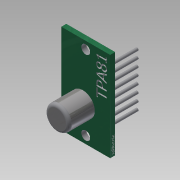
# Autodesk Inventor part: TPA81
Saved by Autodesk Inventor 2015 SP1 (Build 190203100, 203)
## iProperties
Created: 2015-01-28
Part Number: TPA81
Material: Generic
Document SubType Name: Modeling
Designer: Rafi Kurnia Putra
Density: 1 g/cm^3
Appearance: Default
Mass: 1.33618 g
Surface Area: 17.4789 cm^2
Volume: 1.33618 cm^3
Author: Rafi Kurnia Putra
Autodesk Inventor part; units mm, degrees
sketch "Sketch1" plane through (0, 0, 0) normal (0, 1, 0) x (-1, 0, 0)
  line L0 (8.3, 15.2) -> (-8.3, 15.2)
  line L1 (-8.3, 15.2) -> (-8.3, -15.2)
  line L2 (-8.3, -15.2) -> (8.3, -15.2)
  line L3 (8.3, -15.2) -> (8.3, 15.2)
  circle A0 centre (0, -12.66) radius 1.5
  circle A1 centre (0, 12.66) radius 1.5
  circle A2 centre (1, 3.9) radius 4.09
  point P0 (0, 0)
  dimension "d0" = 16.6
  dimension "d1" = 30.4
  dimension "d2" = 3
  dimension "d3" = 3
  dimension "d4" = 2.54
  dimension "d5" = 2.54
  dimension "d6" = 8.18
  dimension "d7" = 7.3
  dimension "d8" = 11.3
  constraints: 8 end point, 3 centre point, 2 parallel, 1 horizontal, 1 perpendicular
  measures "d0" distance of L2.end L1.end
  measures "d1" distance of L1.end L0.end
  measures "d2" diameter of A0
  measures "d3" diameter of A1
  measures "d4" distance from line of A1.centre L0
  measures "d5" distance from line of A0.centre L2
  measures "d6" diameter of A2
  measures "d7" distance from line of A2.centre L3
  measures "d8" distance from line of L0 A2.centre
extrude "Extrusion1" add sketch "Sketch1" along normal blind 1.7
extrude "Extrusion2" add sketch "Sketch1" along normal blind 10.5 contours A2
fillet "Fillet1" radius 1 1 edges at (3.09, 10.5, 3.9)
sketch "Sketch2" plane through (0, 1.7, 0) normal (0, 1, 0) x (1, 0, 0)
  line L0 (3.3822, -3.3689) -> (3.3822, 14.1226) construction
  line L1 (3.3822, 14.1226) -> (7.041, 14.1226) construction
  line L2 (7.041, 14.1226) -> (7.041, -3.3689) construction
  line L3 (7.041, -3.3689) -> (3.3822, -3.3689) construction
  point P0 (0, 0)
  constraints: 2 other
sketch "Sketch3" plane through (0, 0, 0) normal (0, -1, 0) x (1, 0, 0)
  circle A0 centre (5.76, 7.98) radius 0.5
  circle A1 centre (5.76, 5.44) radius 0.5
  circle A2 centre (5.76, 2.9) radius 0.5
  circle A3 centre (5.76, -2.18) radius 0.5
  circle A4 centre (5.76, -4.72) radius 0.5
  circle A5 centre (5.76, -7.26) radius 0.5
  circle A6 centre (5.76, -9.8) radius 0.5
  line L0 (8.3, 15.2) -> (8.3, -15.2) projected
  line L1 (8.3, -15.2) -> (-8.3, -15.2) projected
  circle A7 centre (5.76, 0.36) radius 0.5
  point P0 (0, 0)
  dimension "d30" = 1
  dimension "d31" = 1
  dimension "d32" = 1
  dimension "d33" = 1
  dimension "d34" = 1
  dimension "d35" = 1
  dimension "d36" = 1
  dimension "d37" = 2.54
  dimension "d38" = 2.54
  dimension "d39" = 2.54
  dimension "d40" = 2.54
  dimension "d41" = 2.54
  dimension "d43" = 2.54
  dimension "d44" = 5.4
  dimension "d47" = 1
  dimension "d48" = 2.54
  dimension "d49" = 2.54
  constraints: 8 centre point, 1 vertical alignment
  measures "d30" diameter of A0
  measures "d31" diameter of A1
  measures "d32" diameter of A2
  measures "d33" diameter of A3
  measures "d34" diameter of A4
  measures "d35" diameter of A5
  measures "d36" diameter of A6
  measures "d37" distance of A1.centre A0.centre
  measures "d38" distance of A1.centre A2.centre
  measures "d39" distance of A4.centre A3.centre
  measures "d40" distance of A4.centre A5.centre
  measures "d41" distance of A5.centre A6.centre
  measures "d43" distance from line of A6.centre L0
  measures "d44" distance from line of A6.centre L1
  measures "d47" diameter of A7
  measures "d48" distance of A7.centre A2.centre
  measures "d49" distance of A3.centre A7.centre
extrude "Extrusion3" add sketch "Sketch3" along normal blind 10 contours A0 | A1 | A2 | A3 | A4 | A5 | A6
extrude "Extrusion4" add sketch "Sketch3" along normal blind 10 contours A7
sketch "Sketch4" plane through (0, 1.7, 0) normal (0, 1, 0) x (1, 0, 0)
  line L0 (3.5532, 0.6031) -> (3.5532, 14.2089) construction
  line L1 (3.5532, 14.2089) -> (12.8953, 14.2089) construction
  line L2 (12.8953, 14.2089) -> (12.8953, 0.6031) construction
  line L3 (12.8953, 0.6031) -> (3.5532, 0.6031) construction
  line L4 (7.1326, 1.7745) -> (4.0467, 1.7745)
  line L5 (4.0467, 1.7745) -> (4.0467, 0.6003)
  line L6 (4.0467, 0.6003) -> (3.6326, 0.6003)
  line L7 (3.6326, 0.6003) -> (3.6326, 3.4139)
  line L8 (3.6326, 3.4139) -> (4.0467, 3.4139)
  line L9 (4.0467, 3.4139) -> (4.0467, 2.2397)
  line L10 (4.0467, 2.2397) -> (7.1326, 2.2397)
  line L11 (7.1326, 2.2397) -> (7.1326, 1.7745)
  spline S0 degree 2 poles (4.6877, 5.9807) (4.9146, 5.9807) (5.3231, 5.8191) (5.4649, 5.6744) knots 0 0 0 1 2 2 2
  spline S1 degree 2 poles (5.4649, 5.6744) (5.6436, 5.4929) (5.8279, 5.0022) (5.8279, 4.6278) knots 0 0 0 1 2 2 2
  line L12 (5.8279, 4.6278) -> (5.8279, 4.2336)
  line L13 (5.8279, 4.2336) -> (7.1326, 4.2336)
  line L14 (7.1326, 4.2336) -> (7.1326, 3.7684)
  line L15 (7.1326, 3.7684) -> (3.6326, 3.7684)
  line L16 (3.6326, 3.7684) -> (3.6326, 4.6477)
  spline S2 degree 2 poles (3.6326, 4.6477) (3.6326, 4.9597) (3.7347, 5.3965) (3.851, 5.5638) knots 0 0 0 1 2 2 2
  spline S3 degree 2 poles (3.851, 5.5638) (3.9843, 5.7595) (4.3956, 5.9807) (4.6877, 5.9807) knots 0 0 0 1 2 2 2
  spline S4 degree 2 poles (4.7019, 5.4957) (4.5204, 5.4957) (4.2538, 5.3709) (4.1687, 5.2433) knots 0 0 0 1 2 2 2
  spline S5 degree 2 poles (4.1687, 5.2433) (4.0949, 5.1327) (4.0354, 4.8377) (4.0354, 4.6193) knots 0 0 0 1 2 2 2
  line L17 (4.0354, 4.6193) -> (4.0354, 4.2336)
  line L18 (4.0354, 4.2336) -> (5.4308, 4.2336)
  line L19 (5.4308, 4.2336) -> (5.4308, 4.5512)
  spline S6 degree 2 poles (5.4308, 4.5512) (5.4308, 4.8349) (5.3401, 5.1837) (5.221, 5.2972) knots 0 0 0 1 2 2 2
  spline S7 degree 2 poles (5.221, 5.2972) (5.116, 5.4021) (4.8692, 5.4957) (4.7019, 5.4957) knots 0 0 0 1 2 2 2
  line L20 (7.1326, 6.046) -> (3.6326, 7.2259)
  line L21 (3.6326, 7.2259) -> (3.6326, 7.7988)
  line L22 (3.6326, 7.7988) -> (7.1326, 8.9787)
  line L23 (7.1326, 8.9787) -> (7.1326, 8.488)
  line L24 (7.1326, 8.488) -> (6.1541, 8.1704)
  line L25 (6.1541, 8.1704) -> (6.1541, 6.8345)
  line L26 (6.1541, 6.8345) -> (7.1326, 6.5168)
  line L27 (7.1326, 6.5168) -> (7.1326, 6.046)
  line L28 (5.757, 8.0427) -> (4.1091, 7.501)
  line L29 (4.1091, 7.501) -> (5.757, 6.9621)
  line L30 (5.757, 6.9621) -> (5.757, 8.0427)
  spline S8 degree 2 poles (7.212, 10.2692) (7.212, 10.0083) (7.056, 9.58) (6.9114, 9.4297) knots 0 0 0 1 2 2 2
  spline S9 degree 2 poles (6.9114, 9.4297) (6.7696, 9.2822) (6.3838, 9.129) (6.1654, 9.129) knots 0 0 0 1 2 2 2
  spline S10 degree 2 poles (6.1654, 9.129) (5.8818, 9.129) (5.4053, 9.4325) (5.2635, 9.7218) knots 0 0 0 1 2 2 2
  line L31 (5.2635, 9.7218) -> (5.2493, 9.7218)
  spline S11 degree 2 poles (5.2493, 9.7218) (5.099, 9.4637) (4.7416, 9.2141) (4.475, 9.2141) knots 0 0 0 1 2 2 2
  spline S12 degree 2 poles (4.475, 9.2141) (4.0808, 9.2141) (3.5532, 9.8098) (3.5532, 10.2692) knots 0 0 0 1 2 2 2
  spline S13 degree 2 poles (3.5532, 10.2692) (3.5532, 10.7457) (4.0524, 11.3215) (4.4438, 11.3215) knots 0 0 0 1 2 2 2
  spline S14 degree 2 poles (4.4438, 11.3215) (4.6792, 11.3215) (5.1387, 11.0464) (5.2692, 10.7883) knots 0 0 0 1 2 2 2
  line L32 (5.2692, 10.7883) -> (5.2834, 10.7883)
  spline S15 degree 2 poles (5.2834, 10.7883) (5.4252, 11.0946) (5.8336, 11.4094) (6.1569, 11.4094) knots 0 0 0 1 2 2 2
  spline S16 degree 2 poles (6.1569, 11.4094) (6.6051, 11.4094) (7.212, 10.7571) (7.212, 10.2692) knots 0 0 0 1 2 2 2
  spline S17 degree 2 poles (6.2023, 10.9273) (5.9868, 10.9273) (5.7315, 10.7571) (5.601, 10.516) knots 0 0 0 1 2 2 2
  spline S18 degree 2 poles (5.601, 10.516) (5.5556, 10.4366) (5.4507, 10.17) (5.3826, 10.0026) knots 0 0 0 1 2 2 2
  spline S19 degree 2 poles (5.3826, 10.0026) (5.5103, 9.8098) (5.8903, 9.6027) (6.1314, 9.6027) knots 0 0 0 1 2 2 2
  spline S20 degree 2 poles (6.1314, 9.6027) (6.4491, 9.6027) (6.8632, 9.9856) (6.8632, 10.2749) knots 0 0 0 1 2 2 2
  spline S21 degree 2 poles (6.8632, 10.2749) (6.8632, 10.5699) (6.5086, 10.9273) (6.2023, 10.9273) knots 0 0 0 1 2 2 2
  spline S22 degree 2 poles (4.4495, 10.862) (4.2141, 10.862) (3.8992, 10.5472) (3.8992, 10.2664) knots 0 0 0 1 2 2 2
  spline S23 degree 2 poles (3.8992, 10.2664) (3.8992, 10.0111) (4.18, 9.685) (4.4211, 9.685) knots 0 0 0 1 2 2 2
  spline S24 degree 2 poles (4.4211, 9.685) (4.5941, 9.685) (4.8352, 9.8523) (4.9316, 10.0196) knots 0 0 0 1 2 2 2
  spline S25 degree 2 poles (4.9316, 10.0196) (4.9714, 10.0905) (5.1103, 10.3912) (5.15, 10.5132) knots 0 0 0 1 2 2 2
  spline S26 degree 2 poles (5.15, 10.5132) (4.994, 10.7174) (4.6622, 10.862) (4.4495, 10.862) knots 0 0 0 1 2 2 2
  line L33 (7.1326, 13.8203) -> (7.1326, 12.1128)
  line L34 (7.1326, 12.1128) -> (6.7752, 12.1128)
  line L35 (6.7752, 12.1128) -> (6.7752, 12.7482)
  line L36 (6.7752, 12.7482) -> (4.4296, 12.7482)
  line L37 (4.4296, 12.7482) -> (4.4296, 12.1128)
  line L38 (4.4296, 12.1128) -> (4.1091, 12.1128)
  spline S27 degree 2 poles (4.1091, 12.1128) (4.1091, 12.473) (3.9049, 12.8134) (3.6213, 12.8361) knots 0 0 0 1 2 2 2
  line L39 (3.6213, 12.8361) -> (3.6213, 13.1991)
  line L40 (3.6213, 13.1991) -> (6.7752, 13.1991)
  line L41 (6.7752, 13.1991) -> (6.7752, 13.8203)
  line L42 (6.7752, 13.8203) -> (7.1326, 13.8203)
  point P0 (0, 0)
  constraints: 2 other
sketch "Sketch5" plane through (8.3, 0, 15.2) normal (1, 0, 0) x (0, 0, -1)
  line L0 (0.6114, 1.3065) -> (20.6329, 1.3065) construction
  line L1 (20.6329, 1.3065) -> (20.6329, -2.4459) construction
  line L2 (20.6329, -2.4459) -> (0.6114, -2.4459) construction
  line L3 (0.6114, -2.4459) -> (0.6114, 1.3065) construction
  line L4 (1.1009, 0.8705) -> (1.0944, 0.8705)
  spline S0 degree 2 poles (1.0944, 0.8705) (1.0798, 0.8746) (1.0482, 0.8762) (1.0263, 0.8762) knots 0 0 0 1 2 2 2
  spline S1 degree 2 poles (1.0263, 0.8762) (0.9753, 0.8762) (0.8748, 0.8316) (0.8294, 0.7879) knots 0 0 0 1 2 2 2
  line L5 (0.8294, 0.7879) -> (0.8294, 0.2554)
  line L6 (0.8294, 0.2554) -> (0.703, 0.2554)
  line L7 (0.703, 0.2554) -> (0.703, 1.0058)
  line L8 (0.703, 1.0058) -> (0.8294, 1.0058)
  line L9 (0.8294, 1.0058) -> (0.8294, 0.894)
  spline S2 degree 2 poles (0.8294, 0.894) (0.8983, 0.9556) (1.0012, 1.0058) (1.0498, 1.0058) knots 0 0 0 1 2 2 2
  spline S3 degree 2 poles (1.0498, 1.0058) (1.0693, 1.0058) (1.0887, 1.0042) (1.1009, 1.0018) knots 0 0 0 1 2 2 2
  line L10 (1.1009, 1.0018) -> (1.1009, 0.8705)
  spline S4 degree 2 poles (1.6171, 0.3349) (1.6017, 0.3235) (1.5498, 0.283) (1.5255, 0.2708) knots 0 0 0 1 2 2 2
  spline S5 degree 2 poles (1.5255, 0.2708) (1.4923, 0.253) (1.4299, 0.2344) (1.3731, 0.2344) knots 0 0 0 1 2 2 2
  spline S6 degree 2 poles (1.3731, 0.2344) (1.327, 0.2344) (1.2435, 0.2692) (1.2119, 0.3008) knots 0 0 0 1 2 2 2
  spline S7 degree 2 poles (1.2119, 0.3008) (1.1819, 0.3316) (1.1454, 0.4224) (1.1454, 0.4726) knots 0 0 0 1 2 2 2
  spline S8 degree 2 poles (1.1454, 0.4726) (1.1454, 0.5504) (1.2111, 0.6606) (1.2824, 0.6922) knots 0 0 0 1 2 2 2
  spline S9 degree 2 poles (1.2824, 0.6922) (1.3456, 0.7214) (1.5174, 0.7433) (1.6171, 0.749) knots 0 0 0 1 2 2 2
  line L11 (1.6171, 0.749) -> (1.6171, 0.7733)
  spline S10 degree 2 poles (1.6171, 0.7733) (1.6171, 0.817) (1.5903, 0.8713) (1.566, 0.8867) knots 0 0 0 1 2 2 2
  spline S11 degree 2 poles (1.566, 0.8867) (1.5417, 0.9021) (1.472, 0.9118) (1.4347, 0.9118) knots 0 0 0 1 2 2 2
  spline S12 degree 2 poles (1.4347, 0.9118) (1.391, 0.9118) (1.2727, 0.8859) (1.2135, 0.8608) knots 0 0 0 1 2 2 2
  line L12 (1.2135, 0.8608) -> (1.2062, 0.8608)
  line L13 (1.2062, 0.8608) -> (1.2062, 0.9896)
  spline S13 degree 2 poles (1.2062, 0.9896) (1.2411, 0.9994) (1.3715, 1.0237) (1.4355, 1.0237) knots 0 0 0 1 2 2 2
  spline S14 degree 2 poles (1.4355, 1.0237) (1.5133, 1.0237) (1.6195, 0.9994) (1.6616, 0.9678) knots 0 0 0 1 2 2 2
  spline S15 degree 2 poles (1.6616, 0.9678) (1.703, 0.937) (1.7435, 0.8389) (1.7435, 0.7684) knots 0 0 0 1 2 2 2
  line L14 (1.7435, 0.7684) -> (1.7435, 0.2554)
  line L15 (1.7435, 0.2554) -> (1.6171, 0.2554)
  line L16 (1.6171, 0.2554) -> (1.6171, 0.3349)
  line L17 (1.6171, 0.4402) -> (1.6171, 0.6485)
  spline S16 degree 2 poles (1.6171, 0.6485) (1.5717, 0.6444) (1.4347, 0.6306) (1.3918, 0.6177) knots 0 0 0 1 2 2 2
  spline S17 degree 2 poles (1.3918, 0.6177) (1.3415, 0.6023) (1.2759, 0.5383) (1.2759, 0.4815) knots 0 0 0 1 2 2 2
  spline S18 degree 2 poles (1.2759, 0.4815) (1.2759, 0.4167) (1.3488, 0.3511) (1.4185, 0.3511) knots 0 0 0 1 2 2 2
  spline S19 degree 2 poles (1.4185, 0.3511) (1.4777, 0.3511) (1.5749, 0.4021) (1.6171, 0.4402) knots 0 0 0 1 2 2 2
  line L18 (2.3156, 1.1785) -> (2.3091, 1.1785)
  spline S20 degree 2 poles (2.3091, 1.1785) (2.2921, 1.1849) (2.2289, 1.1963) (2.2038, 1.1963) knots 0 0 0 1 2 2 2
  spline S21 degree 2 poles (2.2038, 1.1963) (2.1244, 1.1963) (2.0563, 1.125) (2.0563, 1.031) knots 0 0 0 1 2 2 2
  line L19 (2.0563, 1.031) -> (2.0563, 1.0058)
  line L20 (2.0563, 1.0058) -> (2.2654, 1.0058)
  line L21 (2.2654, 1.0058) -> (2.2654, 0.9013)
  line L22 (2.2654, 0.9013) -> (2.0603, 0.9013)
  line L23 (2.0603, 0.9013) -> (2.0603, 0.2554)
  line L24 (2.0603, 0.2554) -> (1.9339, 0.2554)
  line L25 (1.9339, 0.2554) -> (1.9339, 0.9013)
  line L26 (1.9339, 0.9013) -> (1.8488, 0.9013)
  line L27 (1.8488, 0.9013) -> (1.8488, 1.0058)
  line L28 (1.8488, 1.0058) -> (1.9339, 1.0058)
  line L29 (1.9339, 1.0058) -> (1.9339, 1.031)
  spline S22 degree 2 poles (1.9339, 1.031) (1.9339, 1.1655) (2.0644, 1.3065) (2.186, 1.3065) knots 0 0 0 1 2 2 2
  spline S23 degree 2 poles (2.186, 1.3065) (2.2208, 1.3065) (2.2881, 1.2992) (2.3156, 1.2943) knots 0 0 0 1 2 2 2
  line L30 (2.3156, 1.2943) -> (2.3156, 1.1785)
  line L31 (2.4874, 0.2554) -> (2.361, 0.2554)
  line L32 (2.361, 0.2554) -> (2.361, 1.0058)
  line L33 (2.361, 1.0058) -> (2.4874, 1.0058)
  line L34 (2.4874, 1.0058) -> (2.4874, 0.2554)
  line L35 (2.4963, 1.1306) -> (2.3529, 1.1306)
  line L36 (2.3529, 1.1306) -> (2.3529, 1.2619)
  line L37 (2.3529, 1.2619) -> (2.4963, 1.2619)
  line L38 (2.4963, 1.2619) -> (2.4963, 1.1306)
  line L39 (3.2945, 0.2554) -> (3.1284, 0.2554)
  line L40 (3.1284, 0.2554) -> (2.8496, 0.6177)
  line L41 (2.8496, 0.6177) -> (2.7994, 0.569)
  line L42 (2.7994, 0.569) -> (2.7994, 0.2554)
  line L43 (2.7994, 0.2554) -> (2.673, 0.2554)
  line L44 (2.673, 0.2554) -> (2.673, 1.3)
  line L45 (2.673, 1.3) -> (2.7994, 1.3)
  line L46 (2.7994, 1.3) -> (2.7994, 0.689)
  line L47 (2.7994, 0.689) -> (3.096, 1.0058)
  line L48 (3.096, 1.0058) -> (3.2532, 1.0058)
  line L49 (3.2532, 1.0058) -> (2.9453, 0.6922)
  line L50 (2.9453, 0.6922) -> (3.2945, 0.2554)
  line L51 (3.9412, 0.2554) -> (3.8148, 0.2554)
  line L52 (3.8148, 0.2554) -> (3.8148, 0.3381)
  spline S24 degree 2 poles (3.8148, 0.3381) (3.7565, 0.287) (3.6519, 0.2344) (3.5871, 0.2344) knots 0 0 0 1 2 2 2
  spline S25 degree 2 poles (3.5871, 0.2344) (3.5385, 0.2344) (3.4518, 0.2668) (3.4202, 0.3016) knots 0 0 0 1 2 2 2
  spline S26 degree 2 poles (3.4202, 0.3016) (3.3877, 0.3365) (3.3521, 0.4426) (3.3521, 0.5188) knots 0 0 0 1 2 2 2
  line L53 (3.3521, 0.5188) -> (3.3521, 1.0058)
  line L54 (3.3521, 1.0058) -> (3.4785, 1.0058)
  line L55 (3.4785, 1.0058) -> (3.4785, 0.578)
  spline S27 degree 2 poles (3.4785, 0.578) (3.4785, 0.518) (3.4874, 0.4394) (3.5028, 0.4102) knots 0 0 0 1 2 2 2
  spline S28 degree 2 poles (3.5028, 0.4102) (3.5182, 0.381) (3.5709, 0.3543) (3.6203, 0.3543) knots 0 0 0 1 2 2 2
  spline S29 degree 2 poles (3.6203, 0.3543) (3.6665, 0.3543) (3.771, 0.407) (3.8148, 0.4451) knots 0 0 0 1 2 2 2
  line L56 (3.8148, 0.4451) -> (3.8148, 1.0058)
  line L57 (3.8148, 1.0058) -> (3.9412, 1.0058)
  line L58 (3.9412, 1.0058) -> (3.9412, 0.2554)
  line L59 (4.5223, 0.8705) -> (4.5158, 0.8705)
  spline S30 degree 2 poles (4.5158, 0.8705) (4.5012, 0.8746) (4.4696, 0.8762) (4.4477, 0.8762) knots 0 0 0 1 2 2 2
  spline S31 degree 2 poles (4.4477, 0.8762) (4.3967, 0.8762) (4.2962, 0.8316) (4.2508, 0.7879) knots 0 0 0 1 2 2 2
  line L60 (4.2508, 0.7879) -> (4.2508, 0.2554)
  line L61 (4.2508, 0.2554) -> (4.1244, 0.2554)
  line L62 (4.1244, 0.2554) -> (4.1244, 1.0058)
  line L63 (4.1244, 1.0058) -> (4.2508, 1.0058)
  line L64 (4.2508, 1.0058) -> (4.2508, 0.894)
  spline S32 degree 2 poles (4.2508, 0.894) (4.3197, 0.9556) (4.4226, 1.0058) (4.4712, 1.0058) knots 0 0 0 1 2 2 2
  spline S33 degree 2 poles (4.4712, 1.0058) (4.4907, 1.0058) (4.5101, 1.0042) (4.5223, 1.0018) knots 0 0 0 1 2 2 2
  line L65 (4.5223, 1.0018) -> (4.5223, 0.8705)
  line L66 (5.2095, 0.2554) -> (5.083, 0.2554)
  line L67 (5.083, 0.2554) -> (5.083, 0.6833)
  spline S34 degree 2 poles (5.083, 0.6833) (5.083, 0.7352) (5.0733, 0.8243) (5.0587, 0.8511) knots 0 0 0 1 2 2 2
  spline S35 degree 2 poles (5.0587, 0.8511) (5.0433, 0.8794) (4.9882, 0.907) (4.9412, 0.907) knots 0 0 0 1 2 2 2
  spline S36 degree 2 poles (4.9412, 0.907) (4.8942, 0.907) (4.7945, 0.8567) (4.7467, 0.8162) knots 0 0 0 1 2 2 2
  line L68 (4.7467, 0.8162) -> (4.7467, 0.2554)
  line L69 (4.7467, 0.2554) -> (4.6203, 0.2554)
  line L70 (4.6203, 0.2554) -> (4.6203, 1.0058)
  line L71 (4.6203, 1.0058) -> (4.7467, 1.0058)
  line L72 (4.7467, 1.0058) -> (4.7467, 0.9224)
  spline S37 degree 2 poles (4.7467, 0.9224) (4.8035, 0.9734) (4.9129, 1.0269) (4.9744, 1.0269) knots 0 0 0 1 2 2 2
  spline S38 degree 2 poles (4.9744, 1.0269) (5.0847, 1.0269) (5.2095, 0.881) (5.2095, 0.7425) knots 0 0 0 1 2 2 2
  line L73 (5.2095, 0.7425) -> (5.2095, 0.2554)
  line L74 (5.5158, 0.2554) -> (5.3894, 0.2554)
  line L75 (5.3894, 0.2554) -> (5.3894, 1.0058)
  line L76 (5.3894, 1.0058) -> (5.5158, 1.0058)
  line L77 (5.5158, 1.0058) -> (5.5158, 0.2554)
  line L78 (5.5247, 1.1306) -> (5.3813, 1.1306)
  line L79 (5.3813, 1.1306) -> (5.3813, 1.2619)
  line L80 (5.3813, 1.2619) -> (5.5247, 1.2619)
  line L81 (5.5247, 1.2619) -> (5.5247, 1.1306)
  spline S39 degree 2 poles (6.1195, 0.3349) (6.1041, 0.3235) (6.0522, 0.283) (6.0279, 0.2708) knots 0 0 0 1 2 2 2
  spline S40 degree 2 poles (6.0279, 0.2708) (5.9947, 0.253) (5.9323, 0.2344) (5.8756, 0.2344) knots 0 0 0 1 2 2 2
  spline S41 degree 2 poles (5.8756, 0.2344) (5.8294, 0.2344) (5.7459, 0.2692) (5.7143, 0.3008) knots 0 0 0 1 2 2 2
  spline S42 degree 2 poles (5.7143, 0.3008) (5.6843, 0.3316) (5.6479, 0.4224) (5.6479, 0.4726) knots 0 0 0 1 2 2 2
  spline S43 degree 2 poles (5.6479, 0.4726) (5.6479, 0.5504) (5.7135, 0.6606) (5.7848, 0.6922) knots 0 0 0 1 2 2 2
  spline S44 degree 2 poles (5.7848, 0.6922) (5.848, 0.7214) (6.0198, 0.7433) (6.1195, 0.749) knots 0 0 0 1 2 2 2
  line L82 (6.1195, 0.749) -> (6.1195, 0.7733)
  spline S45 degree 2 poles (6.1195, 0.7733) (6.1195, 0.817) (6.0928, 0.8713) (6.0684, 0.8867) knots 0 0 0 1 2 2 2
  spline S46 degree 2 poles (6.0684, 0.8867) (6.0441, 0.9021) (5.9744, 0.9118) (5.9372, 0.9118) knots 0 0 0 1 2 2 2
  spline S47 degree 2 poles (5.9372, 0.9118) (5.8934, 0.9118) (5.7751, 0.8859) (5.7159, 0.8608) knots 0 0 0 1 2 2 2
  line L83 (5.7159, 0.8608) -> (5.7086, 0.8608)
  line L84 (5.7086, 0.8608) -> (5.7086, 0.9896)
  spline S48 degree 2 poles (5.7086, 0.9896) (5.7435, 0.9994) (5.874, 1.0237) (5.938, 1.0237) knots 0 0 0 1 2 2 2
  spline S49 degree 2 poles (5.938, 1.0237) (6.0158, 1.0237) (6.1219, 0.9994) (6.1641, 0.9678) knots 0 0 0 1 2 2 2
  spline S50 degree 2 poles (6.1641, 0.9678) (6.2054, 0.937) (6.2459, 0.8389) (6.2459, 0.7684) knots 0 0 0 1 2 2 2
  line L85 (6.2459, 0.7684) -> (6.2459, 0.2554)
  line L86 (6.2459, 0.2554) -> (6.1195, 0.2554)
  line L87 (6.1195, 0.2554) -> (6.1195, 0.3349)
  line L88 (6.1195, 0.4402) -> (6.1195, 0.6485)
  spline S51 degree 2 poles (6.1195, 0.6485) (6.0741, 0.6444) (5.9372, 0.6306) (5.8942, 0.6177) knots 0 0 0 1 2 2 2
  spline S52 degree 2 poles (5.8942, 0.6177) (5.844, 0.6023) (5.7783, 0.5383) (5.7783, 0.4815) knots 0 0 0 1 2 2 2
  spline S53 degree 2 poles (5.7783, 0.4815) (5.7783, 0.4167) (5.8513, 0.3511) (5.921, 0.3511) knots 0 0 0 1 2 2 2
  spline S54 degree 2 poles (5.921, 0.3511) (5.9801, 0.3511) (6.0774, 0.4021) (6.1195, 0.4402) knots 0 0 0 1 2 2 2
  point P0 (15.2, 0)
  constraints: 2 other
extrude "Extrusion5" cut sketch "Sketch5" against normal blind 1
extrude "Extrusion6" cut sketch "Sketch4" against normal blind 1
ref_plane "Work Plane1" through (-1, 0, 0) normal (1, 0, 0) x (0, 1, 0)
sketch "Sketch8" plane through (0, 1.7, 0) normal (0, 1, 0) x (1, 0, 0)
  circle A0 centre (-1, -3.9) radius 4.09 projected
  point P0 (0, 0)
  point P1 (0, 0)
  constraints: 1 coincident
ref_plane "Work Plane2" through (0, 0, 3.9) normal (0, 0, 1) x (1, 0, 0)
sketch "Sketch9" plane through (-8.3, 0, 15.2) normal (0, 0, 1) x (1, 0, 0)
  line L0 (4.21, 10.5) -> (10.39, 10.5) projected
  point P0 (8.3, 0)
ref_plane "Work Plane3" through (0, 10.5, 0) normal (0, 1, 0) x (-1, 0, 0)
sketch "Sketch10" plane through (0, 0, 3.9) normal (0, 0, 1) x (1, 0, 0)
  line L0 (-4.09, 10.5) -> (2.09, 10.5) projected
  line L1 (-1, 10.5) -> (-1, 210.5)
  line L2 (-1, 10.5) -> (199, 10.5) construction
  line L3 (-1, 10.5) -> (-11.4672, 210.2259)
  line L4 (-1, 10.5) -> (199, 10.5) construction
  line L5 (-1, 10.5) -> (9.4672, 210.2259)
  line L6 (-1, 10.5) -> (199, 10.5) construction
  point P0 (0, 0)
  dimension "d59" = 200
  dimension "d60" = 90
  dimension "d61" = 200
  dimension "d62" = 93
  dimension "d63" = 200
  dimension "d64" = 87
  constraints: 12 end point, 3 equal length, 3 horizontal, 1 midpoint, 1 vertical
  measures "d59" distance of L1.start L1.end
  measures "d60" angle of L2 L1
  measures "d61" distance of L1.start L3.end
  measures "d62" angle of L4 L3
  measures "d63" distance of L1.start L5.end
  measures "d64" angle of L6 L5
sketch "Sketch11" plane through (-1, 0, 0) normal (1, 0, 0) x (0, 1, 0)
  line L0 (10.5, 6.99) -> (10.5, 0.81) projected
  line L1 (10.5, 3.9) -> (209.702, -13.9484)
  line L2 (10.5, 3.9) -> (210.5, 3.9) construction
  line L3 (10.5, 3.9) -> (207.3143, -31.6544)
  line L4 (10.5, 3.9) -> (210.5, 3.9) construction
  line L5 (10.5, 3.9) -> (203.3561, -49.0766)
  line L6 (10.5, 3.9) -> (210.5, 3.9) construction
  line L7 (10.5, 3.9) -> (197.8589, -66.0761)
  line L8 (10.5, 3.9) -> (210.5, 3.9) construction
  line L9 (10.5, 3.9) -> (209.702, 21.7484)
  line L10 (10.5, 3.9) -> (207.3143, 39.4544)
  line L11 (10.5, 3.9) -> (203.3561, 56.8766)
  line L12 (10.5, 3.9) -> (197.8589, 73.8761)
  point P0 (0, 0)
  dimension "d65" = 200
  dimension "d66" = 5.12
  dimension "d67" = 200
  dimension "d68" = 10.24
  dimension "d69" = 200
  dimension "d70" = 15.36
  dimension "d71" = 200
  dimension "d72" = 20.48
  constraints: 24 end point, 4 equal length, 4 horizontal, 4 symmetric about line, 1 midpoint
  measures "d65" distance of L1.start L1.end
  measures "d66" angle of L1 L2
  measures "d67" distance of L1.start L3.end
  measures "d68" angle of L3 L4
  measures "d69" distance of L1.start L5.end
  measures "d70" angle of L5 L6
  measures "d71" distance of L1.start L7.end
  measures "d72" angle of L7 L8
body "Solid1"
